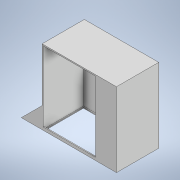
# Autodesk Inventor part: Body_updated
Saved by Autodesk Inventor 2022 (Build 260153000, 153)
## iProperties
Created: 2022-03-29
Part Number: Body_updated
Material: Generic
Document SubType Name: Modeling
Designer: Adit Rambhia
Density: 1 g/cm^3
Appearance: Default
Author: Adit Rambhia
Autodesk Inventor part; units mm, degrees
ref_plane "YZ Plane" through (0, 0, 0) normal (1, 0, 0) x (0, 1, 0)
ref_plane "XZ Plane" through (0, 0, 0) normal (0, 1, 0) x (-1, 0, 0)
ref_plane "XY Plane" through (0, 0, 0) normal (0, 0, 1) x (1, 0, 0)
sketch "Sketch1" plane through (0, 0, 0) normal (0, 0, 1) x (1, 0, 0)
  point P0 (0, 0)
sketch "Sketch2" plane through (0, 0, 0) normal (0, 0, 1) x (1, 0, 0)
  line L0 (0, 0) -> (250, 0)
  line L1 (250, 0) -> (250, 250)
  line L2 (250, 250) -> (0, 250)
  line L3 (0, 250) -> (0, 0)
  line L4 (0, 0) -> (-70, 0)
  line L5 (-70, 0) -> (0, 70)
  dimension "d0" = 250
  dimension "d1" = 250
  dimension "d2" = 70
  dimension "d3" = 45
  constraints: 12 end point, 2 horizontal, 2 parallel, 1 perpendicular, 1 point on line
  measures "d0" distance of L1.end L2.end
  measures "d1" distance of L2.end L0.start
  measures "d2" distance of L0.start L4.end
  measures "d3" angle of L4 L5
extrude "Extrusion1" add sketch "Sketch2" along normal blind 142
sketch "Sketch3" plane through (0, 0, 142) normal (0, 0, 1) x (1, 0, 0)
  line L0 (4, 3) -> (180, 3)
  line L1 (-70, 0) -> (250, 0) projected
  line L2 (4, 3) -> (180, 3) construction
  line L3 (180, 3) -> (180, 246)
  line L4 (4, 3) -> (4, 246)
  line L5 (4, 3) -> (247, 3) construction
  line L6 (250, 250) -> (0, 250) projected
  line L7 (4, 246) -> (180, 246)
  point P0 (0, 0)
  dimension "d6" = 176
  dimension "d7" = 0
  dimension "d8" = 243
  dimension "d9" = 243
  dimension "d10" = 90
  constraints: 12 end point, 2 equal length, 2 horizontal, 1 parallel, 1 perpendicular, 1 vertical
  measures "d6" distance of L0.start L0.end
  measures "d7" distance between parallel lines of L2 L0
  measures "d8" distance of L2.end L3.end
  measures "d9" distance of L0.start L4.end
  measures "d10" angle of L5 L4
extrude "Extrusion2" cut sketch "Sketch3" against normal blind 135
sketch "Sketch4" plane through (4, 3, 142) normal (0, 1, 0) x (1, 0, 0)
  line L0 (3, 3) -> (173, 3)
  line L1 (176, 0) -> (0, 0) projected
  line L2 (173, 3) -> (173, 132)
  line L3 (173, 132) -> (3, 132)
  line L4 (176, 135) -> (0, 135) projected
  line L5 (3, 132) -> (3, 3)
  line L6 (176, 0) -> (176, 135) projected
  line L7 (0, 0) -> (0, 135) projected
  point P0 (-4, 142)
  dimension "d13" = 3
  dimension "d14" = 3
  dimension "d15" = 3
  dimension "d16" = 3
  constraints: 8 end point, 2 parallel, 2 perpendicular
  measures "d13" distance between parallel lines of L4 L3
  measures "d14" distance between parallel lines of L6 L2
  measures "d15" distance between parallel lines of L7 L5
  measures "d16" distance between parallel lines of L1 L0
extrude "Extrusion3" cut sketch "Sketch4" against normal through all contours L5 L3 L2 L0
sketch "Sketch5" plane through (4, 3, 142) normal (0, 1, 0) x (1, 0, 0)
  line L0 (176, 0) -> (0, 0) projected
  line L1 (0, 0) -> (0, 3)
  line L2 (3, 3) -> (3, 132) projected
  line L3 (0, 3) -> (176, 3)
  line L4 (176, 0) -> (176, 135) projected
  line L5 (176, 0) -> (0, 0)
  line L6 (3, 3) -> (173, 3) projected
  point P0 (-4, 142)
  constraints: 6 end point, 2 parallel, 1 perpendicular, 1 point on line
extrude "Extrusion4" add sketch "Sketch5" along normal blind 7
sketch "Sketch6" plane through (-70, 0, 0) normal (0, -1, 0) x (1, 0, 0)
  line L0 (315, 137) -> (254, 137)
  line L1 (254, 137) -> (254, 5)
  line L2 (254, 5) -> (315, 5)
  line L3 (315, 5) -> (315, 137)
  line L4 (0, 142) -> (320, 142) projected
  line L5 (0, 0) -> (320, 0) projected
  line L6 (320, 0) -> (320, 142) projected
  line L7 (247, 139) -> (247, 10) projected
  point P0 (70, 0)
  dimension "d21" = 5
  dimension "d22" = 5
  dimension "d23" = 5
  dimension "d24" = 7
  constraints: 8 end point, 2 parallel, 1 horizontal, 1 perpendicular
  measures "d21" distance between parallel lines of L4 L0
  measures "d22" distance between parallel lines of L5 L2
  measures "d23" distance between parallel lines of L6 L3
  measures "d24" distance between parallel lines of L7 L1
extrude "Extrusion5" cut sketch "Sketch6" against normal blind 246
sketch "Sketch7" plane through (-70, 0, 0) normal (0, -1, 0) x (1, 0, 0)
  line L0 (254, 5) -> (254, 137) projected
  line L1 (315, 137) -> (315, 5) projected
  line L2 (254, 137) -> (315, 137)
  line L3 (315, 137) -> (315, 5)
  line L4 (315, 5) -> (254, 5)
  line L5 (254, 5) -> (254, 137)
  point P0 (70, 0)
  point P1 (315, 5)
  constraints: 8 end point, 2 parallel, 1 horizontal, 1 perpendicular
extrude "Extrusion6" add sketch "Sketch7" against normal blind 10
body "Solid1"
